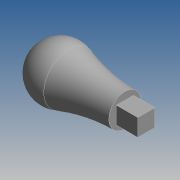
# Autodesk Inventor part: I002
Saved by Autodesk Inventor 2017 (Build 210142000, 142)
## iProperties
Created: 2018-10-05
Part Number: I002
Material: Générique
Document SubType Name: Modeling
Designer: Gilles Mottiez
Density: 1 g/cm^3
Appearance: Par défaut
Description: Pieds
Author: Gilles Mottiez
Autodesk Inventor part; units mm, degrees
ref_plane "YZ Plane" through (0, 0, 0) normal (1, 0, 0) x (0, 1, 0)
ref_plane "XZ Plane" through (0, 0, 0) normal (0, 1, 0) x (-1, 0, 0)
ref_plane "XY Plane" through (0, 0, 0) normal (0, 0, 1) x (1, 0, 0)
sketch "Sketch1" plane through (0, 0, 0) normal (0, 0, 1) x (1, 0, 0)
  line L0 (0, 0) -> (30, 0) construction
  circle A0 centre (0, 0) radius 12.5 construction
  line L1 (0, 7.5) -> (30, 7.5) construction
  arc A1 (4.0541, 11.8243) -> (30, 7.5) centre (30, 87.5) ccw
  line L2 (0, 0) -> (-12.5, 0) construction
  arc A2 (4.0541, 11.8243) -> (-12.5, 0) centre (0, 0) ccw
  line L3 (30, 7.5) -> (30, 0)
  line L4 (-12.5, 0) -> (30, 0)
  dimension "d0" = 30
  dimension "d1" = 25
  dimension "d3" = 7.5
  constraints: 10 end point, 6 point on circle, 3 centre point, 3 tangent, 2 horizontal, 2 vertical alignment, 1 collinear, 1 concentric, 1 parallel, 1 vertical
  measures "d0" distance of L0.start L0.end
  measures "d1" diameter of A0
  measures "d3" distance between parallel lines of L0 L1
revolve "Révolution1" add sketch "Sketch1" angle 360 about axis through (-12.5, 0, 0) along (1, 0, 0)
sketch "Esquisse3" plane through (30, 0, 0) normal (1, 0, 0) x (0, 0, -1)
  circle A0 centre (0, 0) radius 7.5 construction
  line L0 (4, -4) -> (-4, -4)
  line L1 (-4, -4) -> (-4, 4)
  line L2 (-4, 4) -> (4, 4)
  line L3 (4, 4) -> (4, -4)
  line L4 (4, -4) -> (-4, 4) construction
  line L5 (-4, -4) -> (4, 4) construction
  point P0 (0, 0)
  dimension "d8" = 8
  dimension "d9" = 8
  constraints: 12 end point, 2 midpoint, 2 parallel, 1 horizontal, 1 perpendicular
  measures "d8" distance of L1.end L2.end
  measures "d9" distance of L0.end L1.end
extrude "Extrusion2" add sketch "Esquisse3" along normal blind 10
